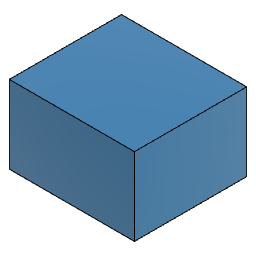
MainBatteryEnclosure v5 (Autodesk Fusion 360 archive; units mm, degrees)
design "Battery Box"
Autodesk Fusion 360 part; units mm, degrees
sketch "Sketch1" plane through (0, 0, 0) normal (0, 0, 1) x (1, 0, 0) in component "Battery Box"
  line L0 (0, 0) -> (184.15, 0)
  line L1 (184.15, 0) -> (184.15, -165.1)
  line L2 (184.15, -165.1) -> (0, -165.1)
  line L3 (0, -165.1) -> (0, 0)
  dimension "d1" = 184.15
  dimension "d2" = 165.1
  constraint horizontal L0
  constraint vertical L1
  constraint horizontal L2
  constraint vertical L3
  constraint coincident L0.start L3.end
  measures "d1" distance of L0.start L0.end
  measures "d2" distance of L0.start L2.end
extrude "Extrude1" add sketch "Sketch1" along normal blind 114.3 in component "Battery Box"
component "Battery Box" placed x (1, 0, 0) y (0, 1, 0) z (0, 0, 1) at (0, 0, 0)

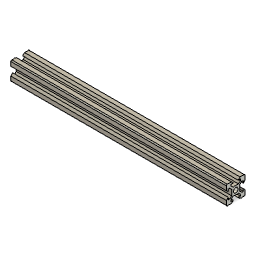
design "Vslot 2020 Sketch v1"
Autodesk Fusion 360 part; units mm, degrees
sketch "Sketch1" plane through (0, 0, 0) normal (0, 1, 0) x (1, 0, 0)
  line L0 (-4.5299, 10) -> (-2.5299, 8)
  line L1 (3, -4.3201) -> (4.9799, -6.3)
  line L2 (6.3, -4.9799) -> (8, -4.9799)
  arc A0 (9, -10) -> (10, -9) centre (9, -9) ccw
  line L3 (-8, 2.5299) -> (-10, 4.5299)
  line L4 (8, -4.9799) -> (8, -2.5299)
  line L5 (-10, -4.5299) -> (-10, -9)
  line L6 (10, 4.5299) -> (8, 2.5299)
  line L7 (-3, 4.3201) -> (3, 4.3201)
  line L8 (-3, -4.3201) -> (3, -4.3201)
  line L9 (4.5299, 10) -> (2.5299, 8)
  line L10 (4.3201, -3) -> (6.3, -4.9799)
  line L11 (8, 4.9799) -> (8, 2.5299)
  line L12 (-9, -10) -> (-4.5299, -10)
  line L13 (-8, -4.9799) -> (-8.0032, -2.5303)
  circle A1 centre (0, 0) radius 2.5
  line L14 (-8, 4.9799) -> (-8, 2.5299)
  line L15 (-4.9799, 6.3) -> (-4.9799, 8)
  line L16 (-4.9799, -6.3) -> (-4.9799, -8)
  line L17 (3, 4.3201) -> (4.9799, 6.3)
  line L18 (4.9799, -8) -> (2.5297, -7.9998)
  line L19 (-4.9799, -8) -> (-2.5299, -8)
  line L20 (-3, 4.3201) -> (-4.9799, 6.3)
  line L21 (4.9799, 6.3) -> (4.9799, 8)
  line L22 (10, -4.5299) -> (10, -9)
  line L23 (4.3201, 3) -> (4.3201, -3)
  line L24 (-4.9799, 8) -> (-2.5299, 8)
  arc A2 (-10, -9) -> (-9, -10) centre (-9, -9) ccw
  line L25 (-10, 4.5299) -> (-10, 9)
  line L26 (-3, -4.3201) -> (-4.9799, -6.3)
  line L27 (-6.3, -4.9799) -> (-8, -4.9799)
  line L28 (-4.5299, 10) -> (-8.1075, 10) construction
  arc A3 (10, 9) -> (9, 10) centre (9, 9) ccw
  line L29 (9, -10) -> (4.5299, -10)
  line L30 (-8.0032, -2.5303) -> (-10, -4.5299)
  line L31 (-4.3201, -3) -> (-6.3, -4.9799)
  line L32 (4.3201, 3) -> (6.3, 4.9799)
  line L33 (10, 4.5299) -> (10, 9)
  line L34 (-4.5299, -10) -> (-2.5299, -8)
  line L35 (10, -4.5299) -> (8, -2.5299)
  line L36 (4.9799, 8) -> (2.5299, 8)
  line L37 (-6.3, 4.9799) -> (-8, 4.9799)
  line L38 (9, 10) -> (4.5299, 10)
  line L39 (4.9799, -6.3) -> (4.9799, -8)
  line L40 (6.3, 4.9799) -> (8, 4.9799)
  arc A4 (-9, 10) -> (-10, 9) centre (-9, 9) ccw
  line L41 (-4.3201, 3) -> (-4.3201, -3)
  line L42 (-9, 10) -> (-4.5299, 10)
  line L43 (4.5299, -10) -> (2.5297, -7.9998)
  line L44 (-4.3201, 3) -> (-6.3, 4.9799)
  dimension "d1" = 5
  dimension "d2" = 6
  dimension "d3" = 2.8
  dimension "d4" = 1.7
  dimension "d5" = 1
  dimension "d8" = 135
  constraint horizontal L29
  constraint horizontal L2
  constraint perpendicular L2 L4
  constraint tangent A0 L22
  constraint tangent A0 L29
  constraint tangent A3 L33
  constraint tangent A3 L38
  constraint equal A0 A3
  constraint tangent A4 L42
  constraint tangent L25 A4
  constraint equal A0 A4
  constraint tangent L5 A2
  constraint equal A0 A2
  constraint horizontal L36
  constraint perpendicular L16 L19
  constraint horizontal L28
  constraint perpendicular L15 L24
  constraint tangent L12 A2
  measures "d1" diameter of A1
  measures "d2" distance of L10.start L23.start
  measures "d3" distance of L10.start L2.start
  measures "d4" distance of L2.start L2.end
  measures "d5" radius of A0
  measures "d8" angle of L0 L28
extrude "Extrude1" add sketch "Sketch1" along normal blind 230
move_body "Move1" bodies 1 to x (0, -1, 0) y (1, 0, 0) z (0, 0, 1) at (-155.0715, 171.0715, 0)
